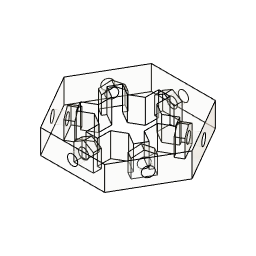
CapacitorJig (Autodesk Fusion 360 design; units mm, degrees)
Autodesk Fusion 360 part; units mm, degrees
sketch "Sketch1" plane through (0, 0, 0) normal (0, 0, 1) x (1, 0, 0)
  line L0 (-5.4993, 9.525) -> (-10.9985, 0)
  line L1 (-10.9985, 0) -> (-5.4993, -9.525)
  line L2 (-5.4993, -9.525) -> (5.4993, -9.525)
  line L3 (5.4993, -9.525) -> (10.9985, 0)
  line L4 (10.9985, 0) -> (5.4993, 9.525)
  line L5 (5.4993, 9.525) -> (-5.4993, 9.525)
  line L6 (-8.386, -14.525) -> (8.386, -14.525)
  line L7 (8.386, -14.525) -> (16.772, 0)
  line L8 (16.772, 0) -> (8.386, 14.525)
  line L9 (8.386, 14.525) -> (-8.386, 14.525)
  line L10 (-8.386, 14.525) -> (-16.772, 0)
  line L11 (-16.772, 0) -> (-8.386, -14.525)
  dimension "d1" = 19.05
  dimension "d2" = 5
  measures "d1" distance of L2 L5
extrude "Extrude1" add sketch "Sketch1" along normal blind 6.35
sketch "Sketch2" plane through (0, 0, 6.35) normal (0, 0, 1) x (-1, 0, 0)
  line L0 (5.4993, -9.525) -> (-5.4993, -9.525)
  line L1 (-5.4993, -9.525) -> (-10.9985, 0)
  line L2 (-10.9985, 0) -> (-5.4993, 9.525)
  line L3 (-5.4993, 9.525) -> (5.4993, 9.525)
  line L4 (5.4993, 9.525) -> (10.9985, 0)
  line L5 (10.9985, 0) -> (5.4993, -9.525)
  line L6 (16.772, 0) -> (8.386, 14.525)
  line L7 (8.386, 14.525) -> (-8.386, 14.525)
  line L8 (-8.386, 14.525) -> (-16.772, 0)
  line L9 (-16.772, 0) -> (-8.386, -14.525)
  line L10 (-8.386, -14.525) -> (8.386, -14.525)
  line L11 (8.386, -14.525) -> (16.772, 0)
  line L12 (1.5, -9.525) -> (1.5, -2.5981)
  line L13 (1.5, -2.5981) -> (7.4989, -6.0615)
  line L14 (1.5, -6.0615) -> (4.4994, -4.3298)
  dimension "d5" = 1.5
  constraint perpendicular L10 L12
  constraint coincident L0 L12.start
  constraint coincident L5 L13.end
  constraint perpendicular L5 L13
  constraint equal L12 L13
  constraint midpoint L13 L14.end
  measures "d5" horizontal distance of origin L12.start
extrude "Extrude2" add sketch "Sketch2" against normal up to surface (6.35 mm away) contours L0 L5 L12 L13 L14
pattern_circular "C-Pattern1" count 6 over 360 about axis through (0, 0, 1.75) along (0, 0, 1) of "Extrude2"
sketch "Sketch3" plane through (0, 14.525, 0) normal (0, 1, 0) x (-1, 0, 0)
  line L0 (-8.386, 0) -> (8.386, 0)
  line L1 (8.386, 0) -> (8.386, 6.35)
  line L2 (8.386, 6.35) -> (-8.386, 6.35)
  line L3 (-8.386, 6.35) -> (-8.386, 0)
  point P0 (0, 3.175)
  point P1 (8.386, 3.175)
  constraint midpoint L1 P1
  constraint horizontal P0 P1
hole "Hole1" at (0, 14.525, 3.175) direction (0, -1, 0) diameter 2.7 end through all
pattern_circular "C-Pattern2" count 3 over 360 about axis through (0, 0, 1.75) along (0, 0, 1) of "Hole1"
sketch "Sketch4" plane through (8.2489, -4.7625, 0) normal (-0.866025, 0.5, 0) x (-0.5, -0.866025, 0)
  circle A0 centre (0, 3.175) radius 1.35
  line L0 (-1.5, 6.35) -> (-1.5, 0)
  line L1 (-1.5, 0) -> (1.5, 0)
  line L2 (1.5, 0) -> (1.5, 6.35)
  line L3 (1.5, 6.35) -> (-1.5, 6.35)
  line L4 (-2.55, 1.7028) -> (0, 0.2305)
  line L5 (0, 0.2305) -> (2.55, 1.7028)
  line L6 (2.55, 1.7028) -> (2.55, 4.6472)
  line L7 (2.55, 4.6472) -> (0, 6.1195)
  line L8 (0, 6.1195) -> (-2.55, 4.6472)
  line L9 (-2.55, 4.6472) -> (-2.55, 1.7028)
  line L10 (-2.55, 1.7028) -> (-2.55, 0)
  line L11 (-2.55, 0) -> (2.55, 0)
  line L12 (2.55, 0) -> (2.55, 1.7028)
  point P0 (0, 3.175)
  dimension "d15" = 5.1
  constraint coincident P0 A0.centre
  constraint vertical L9
  constraint parallel L9 L10
  constraint perpendicular L0 L11
  constraint vertical L12
  measures "d15" distance of L6 L9
extrude "Extrude3" cut sketch "Sketch4" against normal blind 2.1 contours L0 L2 L4 L5 L7 L8 | L0 L4 L8 L9 | L0 L1 L2 L4 L5 L11 | L0 L4 L10 L11 | L2 L5 L6 L7 | L2 L5 L11 L12
pattern_circular "C-Pattern3" count 6 over 360 about axis through (0, 0, 1.75) along (0, 0, 1) of "Extrude3"
